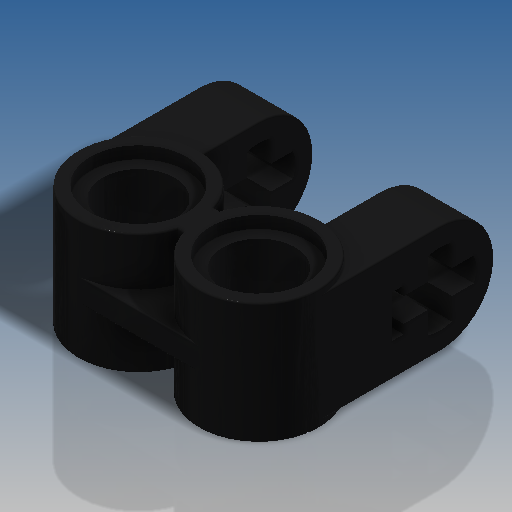
# Autodesk Inventor part: 41678-Black
Saved by Autodesk Inventor 2019.4 (Build 234330000, 330)
## iProperties
Created: 2012-03-28
Part Number: 41678-Black
Document SubType Name: Modeling
Designer: D. Kohfeld
Density: 1.06 g/cm^3
Material: ABS Plastic
Mass: 0.866218 g
Surface Area: 12.1787 cm^2
Volume: 0.817187 cm^3
Appearance: Black
Author: D. Kohfeld
Autodesk Inventor part; units mm, degrees
ref_plane "XZ Plane" through (0, 0, 0) normal (0, 1, 0) x (-1, 0, 0)
ref_plane "XY Plane" through (0, 0, 0) normal (0, 0, 1) x (1, 0, 0)
sketch "Sketch1" plane through (0, 0, 0) normal (0, 0, 1) x (1, 0, 0)
  circle A0 centre (-4, 0) radius 4
  circle A1 centre (4, 0) radius 4
  circle A2 centre (-4, 0) radius 2.4
  circle A3 centre (4, 0) radius 2.4
  circle A4 centre (-4, 0) radius 3.2
  circle A5 centre (4, 0) radius 3.2
  line L0 (-4, 0) -> (4, 0) construction
  line L1 (-4, 4) -> (4, 4)
  line L2 (-4, -4) -> (4, -4)
  line L3 (-0.184243, 1.2) -> (0.184243, 1.2)
  line L4 (-0.184243, -1.2) -> (0.184243, -1.2)
  point P0 (0, 0)
  point P1 (0, 0)
  dimension "d0" = 8
  dimension "d2" = 8
  dimension "d3" = 4.8
  dimension "d4" = 6.4
  dimension "d35" = 2.4
  constraints: 10 end point, 8 point on circle, 6 centre point, 6 coincident, 4 tangent, 3 parallel, 2 equal radius, 2 horizontal, 1 midpoint
  measures "d0" diameter of A0
  measures "d2" distance of point (-4, 0) A1.centre
  measures "d3" diameter of A2
  measures "d4" diameter of A4
  measures "d35" distance between parallel lines of L4 L3
extrude "Extrusion1" add sketch "Sketch1" along normal mid plane 8 contours A0 | A1 L4 A0 | A0 L3 A1 | A1 | A2 | A3 | A4 | A5
extrude "Extrusion13" add sketch "Sketch1" along normal mid plane 1.6 contours A0 L1 A1 L3 | L4 A1 L2 A0
ref_plane "Work Plane1" through (8, 0, 0) normal (1, 0, 0) x (0, 1, 0)
sketch "Sketch3" plane through (8, 0, 0) normal (1, 0, 0) x (0, 1, 0)
  line L0 (-1.2, -4) -> (1.2, -4) construction
  line L1 (1.2, 4) -> (-1.2, 4) construction
  line L2 (4, 0.8) -> (1.2, 0.8) construction
  line L3 (-4, -0.8) -> (-4, 0.8)
  line L4 (-4, -0.8) -> (-1.2, -0.8)
  line L5 (4, -0.8) -> (4, 0.8) construction
  arc A0 (8.8, 2.262742) -> (7.2, 2.262742) centre (8, 0) ccw
  arc A1 (7.2, -2.262742) -> (8.8, -2.262742) centre (8, 0) ccw
  arc A2 (10.262742, -0.8) -> (10.262742, 0.8) centre (8, 0) ccw
  line L6 (10.262742, 0.8) -> (8.8, 0.8)
  line L7 (7.2, 0.8) -> (5.6, 0.8)
  line L8 (8.8, 2.262742) -> (8.8, 0.8)
  line L9 (8.8, -0.8) -> (8.8, -2.262742)
  line L10 (10.262742, -0.8) -> (8.8, -0.8)
  line L11 (7.2, -0.8) -> (5.6, -0.8)
  arc A3 (8, -3.6) -> (8, 3.6) centre (8, 0) ccw
  line L12 (5.6, 0.8) -> (5.6, 1.4)
  line L13 (5.6, 1.4) -> (4.8, 1.4)
  line L14 (4.8, 1.4) -> (4.8, -1.4)
  line L15 (4.8, -1.4) -> (5.6, -1.4)
  line L16 (5.6, -1.4) -> (5.6, -0.8)
  line L17 (0, 3.6) -> (0, -3.6)
  line L18 (0, -3.6) -> (8, -3.6)
  line L19 (0, 3.6) -> (8, 3.6)
  line L20 (7.2, 0.8) -> (7.2, 2.262742)
  line L21 (7.2, -0.8) -> (7.2, -2.262742)
  line L22 (1.2, 0.8) -> (1.2, 4)
  line L23 (-1.2, 4) -> (-1.2, 0.8)
  line L24 (-1.2, 0.8) -> (-4, 0.8)
  line L25 (-1.2, -0.8) -> (-1.2, -4)
  line L26 (1.2, -4) -> (1.2, -0.8)
  line L27 (1.2, -0.8) -> (4, -0.8)
  point P0 (0, 0)
  point P1 (-3.7, 4)
  point P2 (3.7, 4)
  point P3 (3.7, -4)
  point P4 (-3.7, -4)
  point P5 (0, 0)
  point P6 (-4, 4)
  point P7 (4, -4)
  point P8 (4, 4)
  point P9 (-4, -4)
  dimension "d47" = 4.8
  dimension "d49" = 7.2
  dimension "d50" = 0.8
  dimension "d51" = 2.8
  dimension "d52" = 8
  dimension "d53" = 1.6
  constraints: 32 end point, 8 parallel, 8 perpendicular, 8 point on circle, 7 equal length, 4 centre point, 3 tangent, 2 coincident, 2 concentric, 2 horizontal alignment, 2 vertical, 1 collinear, 1 midpoint
  measures "d47" diameter of A1
  measures "d49" diameter of A3
  measures "d50" distance between parallel lines of L14 L16
  measures "d51" distance of L14.start L14.end
  measures "d52" distance from line of A0.centre L17
  measures "d53" distance between parallel lines of L6 L10
extrude "Extrusion4" add sketch "Sketch3" against normal blind 4
mirror "Mirror2" about plane through (0, 0, 0) normal (1, 0, 0) of "Extrusion4"
sketch "Sketch10" plane through (0, 0, 4) normal (0, 0, 1) x (1, 0, 0)
  circle A0 centre (-4, 0) radius 2.4 projected
  circle A1 centre (4, 0) radius 2.4 projected
  circle A2 centre (-4, 0) radius 3.2 projected
  circle A3 centre (4, 0) radius 3.2 projected
  point P0 (0, 0)
extrude "Extrusion14" cut sketch "Sketch10" against normal blind 0.8
mirror "Mirror1" about plane through (0, 0, 0) normal (0, 0, 1) of "Extrusion14"
extrude "Extrusion15" cut sketch "Sketch1" along normal through all both and the other way through all contours A2 | A3
fillet "Fillet1" radius 0.1 24 edges at (-8, 11.6, 0) (-8, 4, 3.6) (-8, 4, -3.6) (8, 11.6, 0) (8, 4, 3.6) (8, 4, -3.6) (4, 6, 3.6) (4, 6, -3.6) (4, 11.6, 0) (-4, 6, 3.6) (-4, 6, -3.6) (-4, 11.6, 0) (-8, 0, 4) (8, 0, 4) (0, -1.2, 4) (0, 1.2, 4) (-8, 0, -4) (8, 0, -4) (0, -4, 0.8) (0, -4, -0.8) (0, 4, 0.8) (0, 4, -0.8) (0, 1.2, -4) (0, -1.2, -4)
equation "\"d0\" = lu"
equation "\"d2\" = lu"
equation "\"d3\" = kd"
equation "\"d4\" = tsd"
equation "\"d7\" = lu"
equation "\"d36\" = wall"
equation "\"d47\" = kd"
equation "\"d49\" = tlad"
equation "\"d52\" = lu"
equation "\"d53\" = axlet"
equation "\"d15\" = 0.5 * lu"
equation "\"d38\" = tsl"
equation "\"d56\" = lf"
equation "\"lu\" = 8"
equation "\"kd\" = 4.8"
equation "\"tsd\" = 6.4"
equation "\"wall\" = 1.6"
equation "\"tlad\" = 7.2"
equation "\"axlet\" = 1.6"
equation "\"tsl\" = 0.8"
equation "\"lf\" = 0.1"
body "Solid1"
